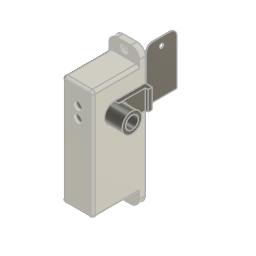
PIR Holder v8 (Autodesk Fusion 360 design; units mm, degrees)
Autodesk Fusion 360 part; units mm, degrees
note: some values were not read from the file. Chosen so that the rebuilt part matches the saved one: which face or edge a step refers to. Set by a fixed rule: which sketch regions a step uses.
sketch "Sketch2" plane through (0, 0, 0) normal (1, 0, 0) x (0, 1, 0) in component "Conn PCB"
  line L0 (-3, 0) -> (-26, 0)
  line L1 (-29, 3) -> (-29, 33.5)
  line L2 (-26, 36.5) -> (-3, 36.5)
  line L3 (0, 33.5) -> (0, 3)
  line L4 (-14.5, 0) -> (-14.5, 3) construction
  line L5 (0, 18.25) -> (-3, 18.25) construction
  line L6 (-3, 33.5) -> (-26, 33.5) construction
  line L7 (-26, 33.5) -> (-26, 3) construction
  line L8 (-26, 3) -> (-3, 3) construction
  line L9 (-3, 3) -> (-3, 33.5) construction
  circle A0 centre (-26, 33.5) radius 1.5
  circle A1 centre (-3, 33.5) radius 1.5
  circle A2 centre (-26, 3) radius 1.5
  circle A3 centre (-3, 3) radius 1.5
  arc A4 (-26, 36.5) -> (-29, 33.5) centre (-26, 33.5) ccw
  arc A5 (0, 33.5) -> (-3, 36.5) centre (-3, 33.5) ccw
  arc A6 (-29, 3) -> (-26, 0) centre (-26, 3) ccw
  arc A7 (-3, 0) -> (0, 3) centre (-3, 3) ccw
  line L10 (-7.5, 7.5) -> (-21.5, 7.5)
  line L11 (-21.5, 7.5) -> (-21.5, 0)
  line L12 (-21.5, 0) -> (-7.5, 0)
  line L13 (-7.5, 0) -> (-7.5, 7.5)
  line L14 (-14.5, 0) -> (-14.5, -4) construction
  line L15 (-10, 10) -> (-19, 10)
  line L16 (-19, 10) -> (-19, -4)
  line L17 (-19, -4) -> (-10, -4)
  line L18 (-10, -4) -> (-10, 10)
  point P0 (-29, 0)
  point P1 (0, 36.5)
  point P2 (-14.5, 3)
  point P3 (-3, 18.25)
  point P4 (-14.5, 0)
  point P5 (-14.5, -4)
  dimension "d11" = 29
  dimension "d12" = 36.5
  dimension "d13" = 3
  dimension "d14" = 3
  dimension "d15" = 3
  dimension "d16" = 3
  dimension "d17" = 3
  dimension "d18" = 3
  dimension "d19" = 3
  dimension "d20" = 3
  dimension "d21" = 3
  dimension "d22" = 3
  dimension "d23" = 23
  dimension "d24" = 30.5
  dimension "d25" = 14
  dimension "d26" = 7.5
  dimension "d27" = 4
  dimension "d28" = 9
  dimension "d29" = 14
  constraint horizontal L0
  constraint vertical L1
  constraint horizontal L2
  constraint vertical L3
  constraint perpendicular L0 L4
  constraint perpendicular L3 L5
  constraint horizontal L6
  constraint vertical L7
  constraint horizontal L8
  constraint vertical L9
  constraint midpoint L8 P2
  constraint coincident P2 L4.end
  constraint midpoint L9 P3
  constraint coincident P3 L5.end
  constraint coincident L6.end L7.start
  constraint coincident L6.start L9.end
  constraint coincident L7.end L8.start
  constraint coincident L8.end L9.start
  constraint tangent L1 A4
  constraint tangent L2 A4
  constraint coincident L3 L5.start
  constraint coincident P1 L2
  constraint coincident P1 L3
  constraint tangent L2 A5
  constraint tangent L3 A5
  constraint coincident L0 L4.start
  constraint coincident P0 L1
  constraint coincident P0 L0
  constraint tangent L1 A6
  constraint tangent L0 A6
  constraint coincident origin L3
  constraint coincident origin L0
  constraint tangent L3 A7
  constraint tangent L0 A7
  constraint horizontal L10
  constraint vertical L11
  constraint horizontal L12
  constraint vertical L13
  constraint midpoint L12 P4
  constraint coincident L4.start L14.start
  constraint coincident P4 L4.start
  constraint vertical L14
  constraint horizontal L15
  constraint vertical L16
  constraint horizontal L17
  constraint vertical L18
  constraint midpoint L17 P5
  constraint coincident P5 L14.end
  measures "d11" distance of origin P0
  measures "d12" distance of origin P1
  measures "d13" distance of L4.start P2
  measures "d14" distance of L5.start P3
  measures "d15" diameter of A0
  measures "d16" diameter of A1
  measures "d17" diameter of A2
  measures "d18" diameter of A3
  measures "d19" radius of A4
  measures "d20" radius of A5
  measures "d21" radius of A6
  measures "d22" radius of A7
  measures "d23" distance of L7.end L8.end
  measures "d24" distance of L6.end L7.end
  measures "d25" distance of L10.start L10.end
  measures "d26" distance of L10.start L12.end
  measures "d27" distance of P4 P5
  measures "d28" distance of L15.start L15.end
  measures "d29" distance of L15.start L17.end
extrude "Extrude1" add sketch "Sketch2" against normal blind 1.6 contours L0 L1 L2 L3 A4 A5 A6 A7 L10 L11 L13 L15 L16 L18 | L0 L10 L12 L13 L18 | L0 L10 L12 L16 L18 | L0 L10 L11 L12 L16 | L10 L15 L16 L18 makes body 1 in component "Conn PCB"
extrude "Extrude2" add sketch "Sketch2" along normal blind 5 contours L0 L10 L12 L13 L18 | L0 L10 L12 L16 L18 | L0 L10 L11 L12 L16 bodies 1 in component "Conn PCB"
extrude "Extrude3" add sketch "Sketch2" against normal blind 11 from surface at -1.6 contours L0 L12 L16 L17 L18 | L0 L10 L12 L16 L18 | L10 L15 L16 L18 bodies 1 in component "Conn PCB"
sketch "Sketch1" plane through (0, 0, 0) normal (1, 0, 0) x (0, 1, 0) in component "PIR PCB"
  line L0 (0, 0) -> (-24, 0)
  line L1 (-24, 0) -> (-24, 33)
  line L2 (-24, 33) -> (0, 33)
  line L3 (0, 33) -> (0, 0)
  line L4 (-12, 33) -> (-12, 30.75) construction
  line L5 (-12, 0) -> (-12, 2.25) construction
  circle A0 centre (-12, 30.75) radius 1
  circle A1 centre (-12, 2.25) radius 1
  circle A2 centre (-12, 16.5) radius 4.15
  line L6 (-12, 33) -> (-12, 0) construction
  line L7 (-24, 33) -> (-22.2, 33) construction
  line L8 (-22.2, 33) -> (-22.2, 23.1) construction
  line L9 (-22.2, 23.1) -> (-22.2, 15.1) construction
  line L10 (-19.5, 26.25) -> (-22.2, 26.25)
  line L11 (-22.2, 26.25) -> (-22.2, 19.95)
  line L12 (-22.2, 19.95) -> (-19.5, 19.95)
  line L13 (-19.5, 19.95) -> (-19.5, 26.25)
  line L14 (-19.5, 18.25) -> (-22.2, 18.25)
  line L15 (-22.2, 18.25) -> (-22.2, 11.95)
  line L16 (-22.2, 11.95) -> (-19.5, 11.95)
  line L17 (-19.5, 11.95) -> (-19.5, 18.25)
  point P0 (-12, 16.5)
  point P1 (-22.2, 23.1)
  point P2 (-22.2, 15.1)
  dimension "d37" = 24
  dimension "d38" = 33
  dimension "d39" = 2.25
  dimension "d40" = 2.25
  dimension "d41" = 2
  dimension "d42" = 2
  dimension "d43" = 8.3
  dimension "d44" = 9.9
  dimension "d45" = 8
  dimension "d46" = 1.8
  dimension "d47" = 2.7
  dimension "d48" = 6.3
  dimension "d49" = 2.7
  dimension "d50" = 6.3
  constraint horizontal L0
  constraint vertical L1
  constraint horizontal L2
  constraint vertical L3
  constraint coincident L0.start L3.end
  constraint midpoint L2 L4.start
  constraint perpendicular L2 L4
  constraint midpoint L0 L5.start
  constraint perpendicular L0 L5
  constraint coincident L4.end A0.centre
  constraint coincident L5.end A1.centre
  constraint midpoint L6 P0
  constraint coincident P0 A2.centre
  constraint coincident L2 L7.end
  constraint perpendicular L1 L7
  constraint perpendicular L2 L8
  constraint parallel L8 L9
  constraint horizontal L10
  constraint vertical L11
  constraint horizontal L12
  constraint vertical L13
  constraint midpoint L11 P1
  constraint coincident P1 L8.end
  constraint horizontal L14
  constraint vertical L15
  constraint horizontal L16
  constraint vertical L17
  constraint midpoint L15 P2
  constraint coincident P2 L9.end
  measures "d37" distance of L0.start L0.end
  measures "d38" distance of L0.start L2.end
  measures "d39" distance of L4.start L4.end
  measures "d40" distance of L5.start L5.end
  measures "d41" diameter of A0
  measures "d42" diameter of A1
  measures "d43" diameter of A2
  measures "d44" distance of L7.end P1
  measures "d45" distance of P1 P2
  measures "d46" distance of L1.end L7.end
  measures "d47" distance of L10.start L10.end
  measures "d48" distance of L10.start L12.end
  measures "d49" distance of L14.start L14.end
  measures "d50" distance of L14.start L16.end
extrude "Extrude1'" add sketch "Sketch1" along normal blind 4.5 separate body contours A2 makes body 2 in component "PIR PCB"
extrude "Extrude2'" add sketch "Sketch1" against normal blind 1.2 contours L0 L1 L2 L3 | A2 | L10 L11 L12 L13 | L14 L15 L16 L17 bodies 2 in component "PIR PCB"
extrude "Extrude3'" add sketch "Sketch1" against normal blind 8 from surface at -1.2 contours L10 L11 L12 L13 | L14 L15 L16 L17 bodies 2 in component "PIR PCB"
sketch "Sketch2 (2)" plane through (0, -22.2, 0) normal (0, -1, 0) x (1, 0, 0) in component "PIR PCB"
  line L0 (-1.2, 19.95) -> (-1.2, 26.25)
  line L1 (-1.2, 26.25) -> (-9.2, 26.25)
  line L2 (-9.2, 26.25) -> (-9.2, 19.95)
  line L3 (-9.2, 19.95) -> (-1.2, 19.95)
  line L4 (-1.2, 11.95) -> (-1.2, 18.25)
  line L5 (-1.2, 18.25) -> (-9.2, 18.25)
  line L6 (-9.2, 18.25) -> (-9.2, 11.95)
  line L7 (-9.2, 11.95) -> (-1.2, 11.95)
  line L8 (-1.2, 15.1) -> (-5.7, 15.1) construction
  line L9 (-1.2, 23.1) -> (-5.7, 23.1) construction
  circle A0 centre (-5.7, 23.1) radius 2.25
  circle A1 centre (-5.7, 15.1) radius 2.25
  dimension "d58" = 4.5
  dimension "d59" = 4.5
  dimension "d60" = 4.5
  dimension "d61" = 4.5
  constraint midpoint L4 L8.start
  constraint perpendicular L4 L8
  constraint midpoint L0 L9.start
  constraint perpendicular L0 L9
  constraint coincident L9.end A0.centre
  constraint coincident L8.end A1.centre
  measures "d58" distance of L8.start L8.end
  measures "d59" distance of L9.start L9.end
  measures "d60" diameter of A0
  measures "d61" diameter of A1
extrude "Extrude4" add sketch "Sketch2 (2)" along normal blind 1.5 contours A0 | A1 bodies 2 in component "PIR PCB"
sketch "Sketch1 (2)" plane through (0, 0, 0) normal (0, 1, 0) x (1, 0, 0) in component "PIR Holder"
  line L0 (0, 0) -> (0, -5) construction
  circle A0 centre (0, -5) radius 1.5
  line L1 (-11, -100) -> (11, -100)
  line L2 (11, -100) -> (11, 0)
  line L3 (11, 0) -> (-11, 0)
  line L4 (-11, 0) -> (-11, -100)
  line L5 (0, -100) -> (0, -95) construction
  circle A1 centre (0, -95) radius 1.5
  dimension "d1" = 5
  dimension "d2" = 3
  dimension "d3" = 22
  dimension "d4" = 100
  dimension "d5" = 5
  dimension "d6" = 3
  constraint coincident L0.start origin
  constraint vertical L0
  constraint coincident L0.end A0.centre
  constraint horizontal L1
  constraint vertical L2
  constraint horizontal L3
  constraint vertical L4
  constraint midpoint L3 L0.start
  constraint midpoint L1 L5.start
  constraint perpendicular L1 L5
  constraint coincident L5.end A1.centre
  measures "d1" distance of L0.start L0.end
  measures "d2" diameter of A0
  measures "d3" distance of L1.start L1.end
  measures "d4" distance of L1.start L3.end
  measures "d5" distance of L5.start L5.end
  measures "d6" diameter of A1
extrude "Extrude1''" add sketch "Sketch1 (2)" against normal blind 4.5 separate body makes body 3 in component "PIR Holder"
fillet "Fillet1" radius 6 4 edges at (11, -2.25, 100) (-11, -2.25, 100) (11, -2.25, 0) (-11, -2.25, 0) on bodies 3 in component "PIR Holder"
sketch "Sketch2 (3)" plane through (-11, 0, 0) normal (-1, 0, 0) x (0, -1, 0) in component "PIR Holder"
  line L0 (0, 6) -> (4.5, 6)
  line L1 (4.5, 6) -> (4.5, 94)
  line L2 (4.5, 94) -> (0, 94)
  line L3 (0, 94) -> (0, 6)
  line L4 (4.5, 94) -> (4.5, 6)
  line L5 (0, 0) -> (0, 15) construction
  line L6 (0, 15) -> (9, 15) construction
  dimension "d64" = 15
  dimension "d65" = 9
  constraint coincident L5.start origin
  constraint parallel L3 L5
  constraint perpendicular L4 L6
  measures "d64" distance of L5.start L5.end
  measures "d65" distance of L5.end L6.end
sketch "Sketch3" plane through (0, 0, 0) normal (1, 0, 0) x (0, 1, 0) in component "PIR Holder"
  line L0 (-32, 50.5) -> (-9, 50.5)
  line L1 (-20.5, 50.5) -> (-20.5, 55.5) construction
  dimension "d76" = 5
  constraint midpoint L0 L1.start
  constraint perpendicular L0 L1
  measures "d76" distance of L1.start L1.end
sketch "Sketch4" plane through (11, 0, 0) normal (1, 0, 0) x (0, 1, 0) in component "PIR Holder"
  line L0 (-4.5, 6) -> (0, 6)
  line L1 (0, 6) -> (0, 94)
  line L2 (0, 94) -> (-4.5, 94)
  line L3 (-4.5, 94) -> (-4.5, 6)
  circle A0 centre (-22.5, 84) radius 1
  circle A1 centre (-22.5, 55.5) radius 1
  line L4 (-10.5, 86.25) -> (-34.5, 86.25)
  line L5 (-34.5, 86.25) -> (-34.5, 53.25)
  line L6 (-34.5, 53.25) -> (-10.5, 53.25)
  line L7 (-10.5, 53.25) -> (-10.5, 86.25)
  line L8 (-27.5, 14) -> (-27.5, 21.5)
  line L9 (-27.5, 21.5) -> (-13.5, 21.5)
  line L10 (-13.5, 21.5) -> (-13.5, 14)
  line L11 (-13.5, 14) -> (-9, 14)
  arc A2 (-9, 14) -> (-6, 17) centre (-9, 17) ccw
  line L12 (-6, 17) -> (-6, 47.5)
  arc A3 (-6, 47.5) -> (-9, 50.5) centre (-9, 47.5) ccw
  line L13 (-9, 50.5) -> (-32, 50.5)
  arc A4 (-32, 50.5) -> (-35, 47.5) centre (-32, 47.5) ccw
  line L14 (-35, 47.5) -> (-35, 17)
  arc A5 (-35, 17) -> (-32, 14) centre (-32, 17) ccw
  line L15 (-32, 14) -> (-27.5, 14)
  circle A6 centre (-32, 17) radius 1.5
  circle A7 centre (-9, 47.5) radius 1.5
  circle A8 centre (-9, 17) radius 1.5
  circle A9 centre (-32, 47.5) radius 1.5
  line L16 (-13.5, 14) -> (-13.5, 21.5)
  line L17 (-13.5, 21.5) -> (-27.5, 21.5)
  line L18 (-27.5, 21.5) -> (-27.5, 14)
  line L19 (-27.5, 14) -> (-13.5, 14)
  line L20 (-16, 14) -> (-25, 14)
  line L21 (-25, 14) -> (-25, 10)
  line L22 (-25, 10) -> (-16, 10)
  line L23 (-16, 10) -> (-16, 14)
  line L24 (-16, 10) -> (-4.5, 10)
  line L25 (-10.5, 86.25) -> (-10.5, 90.25) construction
  line L26 (-10.5, 90.25) -> (-4.5, 90.25)
  line L27 (-4.5, 90.25) -> (-4.5, 10)
  line L28 (-10.5, 90.25) -> (-34.5, 90.25)
  line L29 (-34.5, 90.25) -> (-38.5, 90.25)
  line L30 (-38.5, 90.25) -> (-38.5, 10)
  line L31 (-38.5, 10) -> (-16, 10)
  line L32 (-34.5, 86.25) -> (-34.5, 90.25) construction
  circle A10 centre (-22.5, 69.75) radius 4.15
  circle A11 centre (-22.5, 69.75) radius 4.65
  circle A12 centre (-22.5, 69.75) radius 4.15
  circle A13 centre (-22.5, 84) radius 3
  circle A14 centre (-22.5, 55.5) radius 3
  circle A15 centre (-32, 47.5) radius 3
  circle A16 centre (-9, 47.5) radius 3
  circle A17 centre (-32, 17) radius 3
  circle A18 centre (-9, 17) radius 3
  circle A19 centre (-32, 47.5) radius 1
  circle A20 centre (-9, 47.5) radius 1
  circle A21 centre (-32, 17) radius 1
  circle A22 centre (-9, 17) radius 1
  circle A23 centre (-22.5, 84) radius 0.85
  circle A24 centre (-22.5, 55.5) radius 0.85
  dimension "d82" = 4
  dimension "d83" = 4
  dimension "d84" = 0.5
  dimension "d87" = 6
  dimension "d88" = 6
  dimension "d89" = 6
  dimension "d90" = 6
  dimension "d91" = 6
  dimension "d92" = 6
  dimension "d93" = 2
  dimension "d94" = 2
  dimension "d95" = 2
  dimension "d96" = 2
  dimension "d97" = 1.7
  dimension "d98" = 1.7
  constraint coincident L22.end L23.start
  constraint coincident L3 L24.end
  constraint perpendicular L3 L24
  constraint coincident L4.start L7.end
  constraint perpendicular L4 L25
  constraint coincident L3 L26.end
  constraint perpendicular L3 L26
  constraint perpendicular L25 L28
  constraint perpendicular L25 L29
  constraint perpendicular L22 L30
  constraint perpendicular L21 L31
  constraint coincident L4.end L5.start
  constraint vertical L32
  constraint concentric A0 A13
  constraint concentric A1 A14
  constraint concentric A4 A15
  constraint concentric A3 A16
  constraint concentric A5 A17
  constraint concentric A2 A18
  constraint concentric A15 A19
  constraint concentric A16 A20
  constraint concentric A17 A21
  constraint concentric A18 A22
  constraint concentric A13 A23
  constraint concentric A1 A24
  measures "d82" distance of L4.start L25.end
  measures "d83" distance of L28.end L29.end
  measures "d87" diameter of A13
  measures "d88" diameter of A14
  measures "d89" diameter of A15
  measures "d90" diameter of A16
  measures "d91" diameter of A17
  measures "d92" diameter of A18
  measures "d93" diameter of A19
  measures "d94" diameter of A20
  measures "d95" diameter of A21
  measures "d96" diameter of A22
  measures "d97" diameter of A23
  measures "d98" diameter of A24
  measures "d182" radius of L29.end
extrude "Extrude2''" add sketch "Sketch4" against normal blind 2 contours L3 L11 A2 L12 A3 L13 A4 L14 A5 L15 L19 L21 L23 L24 L26 L27 L28 L29 L30 L31 A15 A16 A17 A18 | L19 L20 L21 L22 L23 L31 | L8 L9 L10 L16 L17 L18 L19 L20 | L8 L9 L10 L11 L12 L13 L14 L15 L16 L17 L18 A15 A16 A17 A18 | A2 A18 | A5 A17 | A3 A16 | A4 A15 | A0 | A1 | L4 L5 L6 L7 A13 A14 | L4 A13 | L4 A13 | L6 A14 | L6 A14 | A6 | A7 | A8 | A9 | A19 | A20 | A21 | A22 | A23 | A24 bodies 3 in component "PIR Holder"
extrude "Extrude3''" add sketch "Sketch4" against normal up to surface (3 mm away) from surface at -2 contours A0 | A1 | L4 A13 | L4 A13 | L6 A14 | L6 A14 bodies 3 in component "PIR Holder"
extrude "Extrude4'" add sketch "Sketch4" against normal up to surface (5.25 mm away) from surface at -2 contours A2 A18 | A5 A17 | A3 A16 | A4 A15 | A6 | A7 | A8 | A9 bodies 3 in component "PIR Holder"
sketch "Sketch5" plane through (11, 0, 0) normal (1, 0, 0) x (0, 1, 0) in component "PIR Holder"
  line L0 (-10.5, 90.25) -> (-34.5, 90.25)
  line L1 (-10.5, 90.25) -> (-4.5, 90.25)
  line L2 (-34.5, 90.25) -> (-38.5, 90.25)
  line L3 (-38.5, 90.25) -> (-38.5, 10)
  line L4 (-38.5, 10) -> (-16, 10)
  line L5 (-16, 10) -> (-4.5, 10)
  line L6 (-16, 12.2) -> (-4.5, 12.2)
  line L7 (-36.3, 12.2) -> (-16, 12.2)
  line L8 (-36.3, 88.05) -> (-36.3, 12.2)
  line L9 (-34.5, 88.05) -> (-36.3, 88.05)
  line L10 (-10.5, 88.05) -> (-34.5, 88.05)
  line L11 (-10.5, 88.05) -> (-4.5, 88.05)
  line L12 (-4.5, 88.05) -> (-4.5, 90.25)
  line L13 (-4.5, 12.2) -> (-4.5, 10)
  line L14 (-4.5, 88.05) -> (-7.5, 88.05) construction
  line L15 (-7.5, 88.05) -> (-7.5, 85.05) construction
  circle A0 centre (-7.5, 85.05) radius 2.5
  circle A1 centre (-7.5, 85.05) radius 0.875
  line L16 (-10, 85.05) -> (-10, 88.05)
  line L17 (-4.5, 88.05) -> (-4.5, 12.2) construction
  line L18 (-7.5, 82.55) -> (-4.5, 82.55)
  line L19 (-4.5, 82.55) -> (-4.5, 88.05)
  dimension "d108" = -2.2
  dimension "d117" = 3
  dimension "d118" = 3
  dimension "d119" = 5
  dimension "d120" = 1.75
  constraint coincident L1.end L12.end
  constraint perpendicular L1 L12
  constraint coincident L5.end L13.end
  constraint perpendicular L5 L13
  constraint midpoint L11 L14.end
  constraint perpendicular L14 L15
  constraint coincident L15.end A0.centre
  constraint concentric A0 A1
  constraint coincident A0 L16.start
  constraint coincident L11 L16.end
  constraint perpendicular L11 L16
  constraint coincident A0 L18.start
  constraint coincident L17 L18.end
  constraint perpendicular L17 L18
  constraint tangent A0 L18
  constraint tangent A0 L16
  measures "d117" distance of L11.end L14.end
  measures "d118" distance of L14.end L15.end
  measures "d119" diameter of A0
  measures "d120" diameter of A1
extrude "Extrude5" add sketch "Sketch5" against normal up to surface (18 mm away) from surface at -2 contours L0 L1 L2 L3 L4 L5 L6 L7 L8 L9 L10 L11 L12 L13 bodies 3 in component "PIR Holder"
sketch "Sketch6" plane through (0, 0, 10) normal (0, 0, -1) x (1, 0, 0) in component "PIR Holder"
  line L0 (11, 4.5) -> (11, 38.5)
  line L1 (11, 38.5) -> (-9, 38.5)
  line L2 (-9, 38.5) -> (-9, 4.5)
  line L3 (-9, 4.5) -> (11, 4.5)
  line L4 (2.15, 16) -> (2.15, 25)
  line L5 (2.15, 25) -> (-8.85, 25)
  line L6 (-8.85, 25) -> (-8.85, 16)
  line L7 (-8.85, 16) -> (2.15, 16)
  line L8 (-9.25, 15.6) -> (2.55, 15.6)
  line L9 (2.55, 15.6) -> (2.55, 25.4)
  line L10 (2.55, 25.4) -> (-9.25, 25.4)
  line L11 (-9.25, 25.4) -> (-9.25, 15.6)
  line L12 (8.75, 27.5) -> (8.75, 13.5)
  line L13 (3.75, 13.5) -> (8.75, 13.5)
  line L14 (3.75, 27.5) -> (8.75, 27.5)
  line L15 (3.75, 13.5) -> (3.75, 27.5)
  line L16 (3.25, 13) -> (3.25, 28)
  line L17 (3.25, 28) -> (9.25, 28)
  line L18 (9.25, 28) -> (9.25, 13)
  line L19 (3.25, 13) -> (9.25, 13)
  line L20 (2.55, 15.6) -> (3.25, 15.6)
  line L21 (2.55, 25.4) -> (3.25, 25.4)
  dimension "d112" = 0.4
  dimension "d160" = -0.5
  constraint coincident L13.start L15.start
  constraint coincident L14.start L15.end
  constraint coincident L16 L20.end
  constraint perpendicular L16 L20
  constraint coincident L16 L21.end
  constraint perpendicular L16 L21
extrude "Extrude6" cut sketch "Sketch6" against normal up to surface (2.2 mm away) contours L2 L8 L9 L10 | L9 L16 L20 L21 | L16 L17 L18 L19 | L4 L5 L6 L7 | L12 L13 L14 L15 bodies 3 in component "PIR Holder"
chamfer "Chamfer3" distance 2.5 angle 45 2 edges at (3.25, -15.6, 11.1) (3.25, -25.4, 11.1) on bodies 3 in component "PIR Holder"
sketch "Sketch1 (3)" plane through (-9, 0, 0) normal (-1, 0, 0) x (0, -1, 0) in component "PIR Holder Lid"
  line L0 (25.4, 12.2) -> (25.4, 10)
  line L1 (25.4, 10) -> (38.5, 10)
  line L2 (38.5, 10) -> (38.5, 90.25)
  line L3 (38.5, 90.25) -> (4.5, 90.25)
  line L4 (4.5, 90.25) -> (4.5, 88.05)
  line L5 (4.5, 88.05) -> (36.3, 88.05)
  line L6 (36.3, 88.05) -> (36.3, 12.2)
  line L7 (36.3, 12.2) -> (25.4, 12.2)
  line L8 (15.6, 10) -> (15.6, 12.2)
  line L9 (15.6, 12.2) -> (4.5, 12.2)
  line L10 (4.5, 12.2) -> (4.5, 10)
  line L11 (4.5, 10) -> (15.6, 10)
  circle A0 centre (7.5, 85.05) radius 0.875
  circle A1 centre (32, 17) radius 1.5
  line L12 (4.5, 90.25) -> (38.5, 90.25)
  line L13 (38.5, 90.25) -> (38.5, 10)
  line L14 (38.5, 10) -> (4.5, 10)
  line L15 (4.5, 10) -> (4.5, 90.25)
  line L16 (5, 10) -> (5, 90.25)
  circle A2 centre (7.5, 85.05) radius 1
  circle A3 centre (32, 17) radius 1
  line L17 (5, 88.05) -> (36.3, 88.05) construction
  line L18 (36.3, 88.05) -> (36.3, 12.2) construction
  line L19 (36.3, 12.2) -> (5, 12.2) construction
  line L20 (5, 87.55) -> (35.8, 87.55)
  line L21 (35.8, 87.55) -> (35.8, 12.7)
  line L22 (35.8, 12.7) -> (5, 12.7)
  line L23 (25, 24) -> (16, 24)
  line L24 (16, 24) -> (16, 10)
  line L25 (16, 10) -> (25, 10)
  line L26 (25, 10) -> (25, 24)
  line L27 (15, 25) -> (15, 9)
  line L28 (15, 9) -> (26, 9)
  line L29 (26, 9) -> (26, 25)
  line L30 (26, 25) -> (15, 25)
  point P0 (32, 17)
  dimension "d121" = 0.5
  dimension "d122" = 2
  dimension "d124" = 2
  dimension "d126" = 0.5
  dimension "d131" = 1
  constraint coincident L3.end L4.start
  constraint coincident L2.end L3.start
  constraint coincident L1.end L2.start
  constraint coincident L10.end L11.start
  constraint concentric A0 A2
  constraint concentric A1 A3
  constraint coincident L5 L17.start
  constraint coincident L16 L17.start
  constraint coincident L5.end L6.start
  constraint coincident L6.end L7.start
  constraint coincident L9 L19.end
  constraint coincident L16 L19.end
  measures "d122" diameter of A2
  measures "d124" diameter of A3
extrude "Extrude1'''" add sketch "Sketch1 (3)" along normal up to surface (2 mm away) separate body contours L0 L1 L7 L14 L29 | L0 L7 L14 L22 L26 L29 | L5 L6 L7 L16 L20 L21 L22 L29 | L1 L2 L3 L5 L6 L7 L12 L13 L14 L16 L29 | L14 L22 L24 L25 L26 | L16 L20 L21 L22 L27 L29 L30 | L22 L23 L24 L26 L27 L29 L30 | L8 L9 L14 L22 L24 L27 | L22 L23 L24 L26 | L8 L9 L11 L14 L27 | L9 L11 L14 L16 L27 | L9 L16 L22 L27 | A1 makes body 4 in component "PIR Holder Lid"
extrude "Extrude2'''" add sketch "Sketch1 (3)" against normal blind 2 contours L16 L20 L21 L22 L27 L29 L30 | A1 bodies 4 in component "PIR Holder Lid"
chamfer "Chamfer1" distance 1.5 angle 45 2 edges at (-11, -6.5677, 84.6884) (-11, -31.0677, 16.6384) on bodies 4 in component "PIR Holder Lid"
fillet "Fillet2" radius 2 2 edges at (-10, -38.5, 10) (-10, -38.5, 90.25) on bodies 4 in component "PIR Holder Lid"
fillet "Fillet3" radius 2 5 edges at (-11, -20.75, 90.25) (-11, -37.9142, 89.6642) (-11, -38.5, 50.125) (-11, -37.9142, 10.5858) (-11, -20.75, 10) on bodies 4 in component "PIR Holder Lid"
fillet "Fillet2'" radius 2 2 edges at (1, -38.5, 10) (1, -38.5, 90.25) on bodies 3 in component "PIR Holder"
fillet "Fillet3'" radius 2 5 edges at (11, -20.5, 90.25) (11, -37.9142, 89.6642) (11, -38.5, 50.125) (11, -37.9142, 10.5858) (11, -20.5, 10) on bodies 3 in component "PIR Holder"
extrude "Extrude7" add sketch "Sketch5" against normal up to surface (18 mm away) contours L11 A0 L16 L18 L19 | A0 bodies 3 in component "PIR Holder"
sketch "Sketch7" plane through (-7, 0, 0) normal (1, 0, 0) x (0, 1, 0) in component "PIR Holder"
  circle A0 centre (-32, 17) radius 1
  circle A1 centre (-7.5, 85.05) radius 1
  line L0 (-26, 12.7) -> (-26, 25)
  line L1 (-26, 25) -> (-15, 25)
  line L2 (-15, 25) -> (-15, 12.7)
  line L3 (-15, 12.7) -> (-5, 12.7)
  line L4 (-5, 12.7) -> (-5, 87.55)
  line L5 (-5, 87.55) -> (-35.8, 87.55)
  line L6 (-35.8, 87.55) -> (-35.8, 12.7)
  line L7 (-35.8, 12.7) -> (-26, 12.7)
  arc A2 (-36.5, 90.25) -> (-38.5, 88.25) centre (-36.5, 88.25) ccw
  line L8 (-38.5, 88.25) -> (-38.5, 12)
  arc A3 (-38.5, 12) -> (-36.5, 10) centre (-36.5, 12) ccw
  line L9 (-36.5, 10) -> (-5, 10)
  line L10 (-5, 10) -> (-5, 12.7)
  line L11 (-5, 12.7) -> (-15, 12.7)
  line L12 (-15, 12.7) -> (-15, 25)
  line L13 (-15, 25) -> (-26, 25)
  line L14 (-26, 25) -> (-26, 12.7)
  line L15 (-26, 12.7) -> (-35.8, 12.7)
  line L16 (-35.8, 12.7) -> (-35.8, 87.55)
  line L17 (-35.8, 87.55) -> (-5, 87.55)
  line L18 (-5, 87.55) -> (-5, 90.25)
  line L19 (-5, 90.25) -> (-36.5, 90.25)
  circle A4 centre (-32, 17) radius 2.75
  line L20 (-36.3, 88.05) -> (-36.3, 12.2)
  line L21 (-36.3, 12.2) -> (-16, 12.2)
  line L22 (-32, 19.75) -> (-36.3, 19.75)
  line L23 (-29.25, 17) -> (-29.25, 12.2)
  circle A5 centre (-32, 17) radius 0.75
  dimension "d145" = 5.5
  dimension "d162" = -0.25
  constraint concentric A0 A4
  constraint coincident A4 L22.start
  constraint coincident L20 L22.end
  constraint perpendicular L20 L22
  constraint coincident A4 L23.start
  constraint coincident L21 L23.end
  constraint perpendicular L21 L23
  constraint tangent A4 L23
  constraint tangent A4 L22
  measures "d145" diameter of A4
ref_plane "WorkPlane1" through (1.75, -32, 17) normal (-1, 0, 0) x (0, 0, 1) in component "PIR Holder"
sketch "Sketch8" plane through (1.75, -32, 17) normal (-1, 0, 0) x (0, 1, 0) in component "PIR Holder"
  line L0 (-4.3, 4.8) -> (16, 4.8)
  line L1 (-4.3, -71.05) -> (-4.3, 4.8)
  circle A0 centre (-4.3, 4.8) radius 1
  dimension "d150" = 2
  constraint coincident L0.start L1.end
  measures "d150" diameter of A0
extrude "Extrude9" add sketch "Sketch7" along normal blind 3 contours A0 | L6 L7 L15 L16 L20 L21 L22 L23 | L6 L7 L15 L16 A4 L22 L23 | A4 | A5 bodies 3 in component "PIR Holder"
loft "Loft1" add profiles "Sketch8" section 1 contours L0 L1 A0 picked at (-3.8298, 4.3298) section 2 face at (-4, -31.6, 13.8) on bodies 3 bodies 3 in component "PIR Holder"
extrude "Extrude10" cut sketch "Sketch7" along normal blind 2 contours A5 bodies 3 in component "PIR Holder"
sketch "Sketch9" plane through (0, -38.5, 0) normal (0, -1, 0) x (1, 0, 0) in component "PIR Holder"
  line L0 (9, 12) -> (9, 88.25)
  line L1 (9, 88.25) -> (-9, 88.25)
  line L2 (-9, 88.25) -> (-9, 12)
  line L3 (-9, 12) -> (9, 12)
  circle A0 centre (0.3, 76.35) radius 2.25
  circle A1 centre (0.3, 68.35) radius 2.25
  circle A2 centre (0.3, 76.35) radius 3.25
  circle A3 centre (0.3, 68.35) radius 3.25
  dimension "d155" = 1
  dimension "d156" = 1
extrude "Extrude11" cut sketch "Sketch9" against normal up to surface (2.2 mm away) contours A0 | A1 | A2 | A3 bodies 3 in component "PIR Holder"
chamfer "Chamfer2" distance 2 angle 45 2 edges at (-1.3985, -4.5, 5.5424) (-1.3985, -4.5, 95.5424) on bodies 3 in component "PIR Holder"
ref_plane "WorkPlane1" through (0, 0, 50) normal (0, 1, 0) x (1, 0, 0) in component "Kitchen Baffle"
sketch "Sketch1 (4)" plane through (0, 0, 0) normal (0, 1, 0) x (1, 0, 0) in component "Kitchen Baffle"
  circle A0 centre (0, -5) radius 1.5
  circle A1 centre (0, -95) radius 1.5
  arc A2 (-5, 0) -> (-11, -6) centre (-5, -6) ccw
  line L0 (-11, -6) -> (-11, -94)
  arc A3 (-11, -94) -> (-5, -100) centre (-5, -94) ccw
  line L1 (-5, -100) -> (5, -100)
  arc A4 (5, -100) -> (11, -94) centre (5, -94) ccw
  line L2 (11, -94) -> (11, -6)
  arc A5 (11, -6) -> (5, 0) centre (5, -6) ccw
  line L3 (5, 0) -> (-5, 0)
  line L4 (0, -95) -> (67, -95) construction
  line L5 (11, -65.1) -> (11, -74.4)
  dimension "d164" = 67
  constraint coincident A1.centre L4.start
  constraint perpendicular L2 L4
  measures "d164" distance of A1.centre L4.end
ref_plane "WorkPlane2" through (11, -18.25, 50) normal (1, 0, 0) x (0, 0, 1) in component "Kitchen Baffle"
sketch "Sketch2 (4)" plane through (11, 0, 0) normal (1, 0, 0) x (0, 1, 0) in component "Kitchen Baffle"
  line L0 (-4.5, 12) -> (-4.5, 6)
  line L1 (-4.5, 6) -> (0, 6)
  line L2 (0, 6) -> (0, 94)
  line L3 (0, 94) -> (-4.5, 94)
  line L4 (-4.5, 94) -> (-4.5, 88.25)
  line L5 (-4.5, 88.25) -> (-36.5, 88.25)
  line L6 (-36.5, 88.25) -> (-36.5, 12)
  line L7 (-36.5, 12) -> (-4.5, 12)
  circle A0 centre (-22.5, 69.75) radius 4.65
  line L8 (-22.5, 69.75) -> (-22.5, 94) construction
  line L9 (0, 95, 56) -> (-22.5, 94, 0) construction
  line L10 (-22.5, 69.75) -> (-36.5, 69.75) construction
  point P0 (0, 95)
  constraint coincident A0.centre L8.start
  constraint perpendicular L3 L8
  constraint coincident L6 L10.end
  constraint perpendicular L6 L10
ref_plane "WorkPlane3" through (11, -29.5, 69.75) normal (0, 0, 1) x (0, -1, 0) in component "Kitchen Baffle"
sketch "Sketch3 (2)" plane through (0, 0, 69.75) normal (0, 0, 1) x (1, 0, 0) in component "Kitchen Baffle"
  line L0 (11, -27.15) -> (11, -17.85)
  line L1 (11, -22.5) -> (23.7758, -17.85) construction
  line L2 (11, -22.5) -> (17.8398, -22.5) construction
  line L3 (11, -17.85) -> (23.7758, -17.85)
  line L4 (11, -17.85) -> (11, -15.35)
  line L5 (11, -15.35) -> (23.7758, -15.35)
  line L6 (23.7758, -15.35) -> (23.7758, -17.85)
  point P0 (11, -22.5)
  dimension "d167" = 20
  dimension "d169" = 2.5
  constraint horizontal L2
  constraint coincident P0 L1.start
  constraint coincident L0.end L3.start
  constraint perpendicular L0 L3
  constraint perpendicular L3 L4
  constraint perpendicular L4 L5
  constraint perpendicular L5 L6
  measures "d167" angle of L1 L2
  measures "d169" distance of L0.end L4.end
revolve "Revolve1" add sketch "Sketch3 (2)" angle 360 about axis through (11, -22.5, 69.75) along (1, 0, 0) separate body makes body 5 in component "Kitchen Baffle"
sketch "Sketch4 (2)" plane through (11, 0, 0) normal (1, 0, 0) x (0, 1, 0) in component "Kitchen Baffle"
  circle A0 centre (-22.5, 69.75) radius 7.15
  circle A1 centre (-22.5, 69.75) radius 4.65
  line L0 (-22.5, 69.75) -> (-22.5, 62.6) construction
  line L1 (-22.5, 69.75) -> (-17.85, 69.75)
  line L2 (-22.5, 69.75) -> (-22.5, 76.9) construction
  line L3 (0, 6) -> (0, 94)
  line L4 (-22.5, 62.6) -> (0, 62.6)
  line L5 (-22.5, 76.9) -> (0, 76.9)
  line L6 (-22.5, 76.9) -> (-22.5, 74.4)
  line L7 (-22.5, 62.6) -> (-22.5, 65.1)
  line L8 (0, 62.6) -> (22.5, 62.6)
  line L9 (22.5, 62.6) -> (22.5, 95.7669)
  line L10 (17.5, 100.7669) -> (5, 100.7669)
  line L11 (0, 95.7669) -> (0, 62.6)
  line L12 (0, 95) -> (22.5, 95) construction
  circle A2 centre (11.25, 95) radius 1.5
  line L13 (-3, 62.6) -> (-3, 76.9)
  arc A3 (5, 100.7669) -> (0, 95.7669) centre (5, 95.7669) ccw
  arc A4 (22.5, 95.7669) -> (17.5, 100.7669) centre (17.5, 95.7669) ccw
  point P0 (0, 100)
  point P1 (0, 94)
  point P2 (11.25, 95)
  dimension "d173" = 22.5
  dimension "d174" = 1
  dimension "d175" = 3
  dimension "d176" = 3
  dimension "d182" = 5
  dimension "d183" = 5
  constraint coincident A0.centre A1.centre
  constraint coincident A0 L0.end
  constraint perpendicular L0 L1
  constraint coincident A0 L2.end
  constraint parallel L0 L2
  constraint coincident L3 L4.end
  constraint tangent A0 L4
  constraint coincident L3 L5.end
  constraint perpendicular L3 L5
  constraint coincident A1 L6.end
  constraint coincident L2 L6.end
  constraint coincident A1 L7.end
  constraint coincident L0 L7.end
  constraint horizontal L8
  constraint vertical L9
  constraint horizontal L10
  constraint vertical L11
  constraint coincident L11 L12.start
  constraint coincident L9 L12.end
  constraint perpendicular L9 L12
  constraint coincident L4 L13.start
  constraint coincident L5 L13.end
  constraint perpendicular L5 L13
  constraint tangent L11 A3
  constraint tangent L10 A3
  constraint tangent L9 A4
  constraint tangent L10 A4
  constraint coincident L10 L9.end
  constraint midpoint L12 P2
  constraint coincident P2 A2.centre
  measures "d173" distance of L4.end L8.end
  measures "d174" distance of L12 P1
  measures "d175" diameter of A2
  measures "d176" distance of L4.end L13.start
  measures "d182" radius of A3
  measures "d183" radius of A4
extrude "Extrude1''''" add sketch "Sketch4 (2)" along normal blind 3 contours A0 A1 L6 L7 | A0 L4 L5 L13 | L3 L4 L5 L11 L13 picked at (-21.9402, 76.0266) bodies 5 in component "Kitchen Baffle"
extrude "Extrude2''''" add sketch "Sketch4 (2)" along normal blind 0.5 contours L3 L8 L9 L10 L11 A3 A4 bodies 5 in component "Kitchen Baffle"
extrude "Extrude3'''" add sketch "Sketch4 (2)" along normal blind 2 from surface at 3 contours L3 L4 L5 L11 L13 bodies 5 in component "Kitchen Baffle"
component "Conn PCB" placed x (1, 0, 0) y (0, 1, 0) z (0, 0, 1) at (3.75, -6, 14)
component "PIR PCB" placed x (1, 0, 0) y (0, 1, 0) z (0, 0, 1) at (6, -10.5, 53.25)
component "PIR Holder" placed x (1, 0, 0) y (0, 1, 0) z (0, 0, 1) at (0, 0, 0)
component "PIR Holder Lid" placed x (1, 0, 0) y (0, 1, 0) z (0, 0, 1) at (0, 0, 0)
component "Kitchen Baffle" placed x (1, 0, 0) y (0, 1, 0) z (0, 0, 1) at (0, 0, 0)
named bodies: "PIR Holder", "PIR PCB", "PIR Holder Lid", "PIR Baffle"
